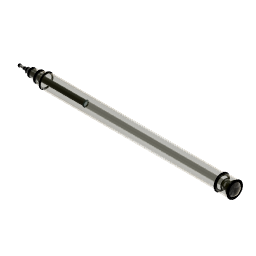
Pen_Model (Autodesk Fusion 360 design; units mm, degrees)
Autodesk Fusion 360 part; units mm, degrees
sketch "Sketch1" plane through (0, 0, 0) normal (0, 1, 0) x (1, 0, 0)
  line L0 (-51.000001, 0) -> (8, 0)
  line L1 (-50.999999, -0.45) -> (-51.000001, -0.5)
  line L2 (-51.000001, -0.5) -> (-48.500001, -0.5)
  line L3 (-48.500001, -0.5) -> (-47.077309, -0.848455)
  line L4 (-47.077309, -0.848455) -> (-47.077309, -0.95)
  line L5 (-41.000001, -1.35) -> (-41.000001, -1.175)
  arc A0 (-51.349999, 0) -> (-50.999999, -0.45) centre (-50.867104, 0.014474) ccw
  line L6 (-51.349999, 0) -> (-51.000001, 0)
  line L7 (-41.000001, -1.35) -> (-44.999999, -1.35)
  line L8 (-44.999999, -1.35) -> (-44.999999, -1.7)
  line L9 (-47.077309, -0.95) -> (-45.299999, -1.537888)
  line L10 (-45.299999, -1.537888) -> (-45.299999, -1.7)
  line L11 (-44.999999, -1.7) -> (-45.299999, -1.7)
  line L12 (-41.000001, -1.175) -> (19, -1.175)
  line L13 (19, -1.175) -> (19, 0)
  line L14 (19, 0) -> (8, 0)
  line L15 (-41.000001, -1.175) -> (-41.000001, 0)
  line L16 (-28.417661, -1.175) -> (-28.417661, 0)
  constraint horizontal L0
  constraint perpendicular L0 L1
  constraint perpendicular L1 L2
  constraint perpendicular L2 L4
  constraint parallel L0 L6
  constraint perpendicular L10 L11
  constraint perpendicular L12 L13
  constraint perpendicular L0 L15
revolve "Revolve1" add sketch "Sketch1" angle 360 about axis through (-51.000001, 0, 0) along (1, 0, 0) makes body 1
move_face "OffsetFaces1" offset -39 1 faces at (19, 0.344804, 0.639991) on bodies 1
sketch "Sketch2" plane through (-20, 0, 0) normal (1, 0, 0) x (0, 1, 0)
  circle A0 centre (0, 0) radius 1.175
sketch "Sketch3" plane through (-20, 0, 0) normal (1, 0, 0) x (0, 1, 0)
  circle A0 centre (0, 0) radius 1.173456
  circle A1 centre (0, 0) radius 1.111334
  constraint coincident A0.centre A1.centre
extrude "Extrude1" add sketch "Sketch3" along normal blind 69 bodies 1
fillet "Fillet1" radius 0.495 1 edges at (-51.000001, -0.180808, -0.466164) on bodies 1
sketch "Sketch4" plane through (0, 0, 0) normal (0, 1, 0) x (1, 0, 0)
  line L0 (-44.999999, -1.35) -> (-44.999999, -1.8)
  line L1 (-44.999999, -1.8) -> (-42.726678, -2.455447)
  line L2 (-42.726678, -2.455447) -> (-42.399999, -2.455447)
  line L3 (-42.399999, -2.455447) -> (-40.838311, -2.905716)
  line L4 (-40.838311, -2.905716) -> (43.000001, -2.905716)
  line L5 (43.000001, -2.905716) -> (43.000001, -3.5)
  line L6 (43.000001, -3.5) -> (49.000001, -3.5)
  line L7 (49.000001, -3.5) -> (49.000001, -1)
  line L8 (49.425851, -1) -> (49.425851, -3.5)
  line L9 (49.425851, -3.5) -> (49.000001, -3.5)
  line L10 (45.000001, 0) -> (45.000001, -2)
  line L11 (45.000001, -2) -> (48.000001, -2)
  line L12 (48.000001, -2) -> (48.000001, -2.6)
  line L13 (48.000001, -2.6) -> (49.000001, -2.6)
  line L14 (49.425851, 0) -> (49.425851, -1)
  arc A0 (49.425851, -2.989421) -> (50.690361, 0.022081) centre (46.648918, -0.052175) ccw
  line L15 (49, -1.173456) -> (49, 1.173456)
  line L16 (-20, 1.173456) -> (-20, -1.173456)
  line L17 (45.000001, 0) -> (45.000001, -2)
  line L18 (49.000001, 0) -> (50.690706, 0)
  line L19 (49.000001, 0) -> (49.000001, -2.6)
  line L20 (49.000001, 0) -> (45.000001, 0)
  constraint vertical L0
  constraint horizontal L2
  constraint parallel L1 L3
  constraint parallel L2 L4
  constraint perpendicular L4 L5
  constraint perpendicular L5 L6
  constraint perpendicular L6 L7
  constraint perpendicular L6 L8
  constraint perpendicular L7 L9
  constraint perpendicular L10 L11
  constraint perpendicular L11 L12
  constraint perpendicular L7 L13
  constraint perpendicular L13 L19
  constraint perpendicular L10 L20
revolve "Revolve2" add sketch "Sketch4" angle 360 about axis through (49.000001, 0, 0) along (1, 0, 0) separate body makes body 2
sketch "Sketch5" plane through (0, 0, 0) normal (0, 1, 0) x (1, 0, 0)
  line L0 (-20, 1.175) -> (-20, -1.175)
  line L1 (-41.000001, 1.175) -> (-41.000001, -1.175)
  line L2 (-41.000001, 1.35) -> (-41.000001, -1.35)
  line L3 (-44.999999, 1.35) -> (-44.999999, -1.35)
  line L4 (49, -1.173456) -> (49, 1.173456)
  line L5 (-20, 1.173456) -> (-20, -1.173456)
  line L6 (49.425851, 2.989421) -> (49.425851, -2.989421)
  line L7 (49.000001, 3.5) -> (49.000001, -3.5)
  line L8 (49.425851, 3.5) -> (49.425851, -3.5)
  line L9 (49.425851, 3.5) -> (49.425851, -3.5)
  line L10 (49.000001, 3.5) -> (49.000001, -3.5)
  line L11 (49.000001, 2.6) -> (49.000001, -2.6)
  line L12 (48.000001, 2.6) -> (48.000001, -2.6)
  line L13 (48.000001, 2) -> (48.000001, -2)
  line L14 (45.000001, 2) -> (45.000001, -2)
  line L15 (-44.999999, 1.7) -> (-44.999999, -1.7)
  line L16 (-45.299999, 1.7) -> (-45.299999, -1.7)
  line L17 (-44.999999, -1.7) -> (-44.999999, -1.73)
  line L18 (-44.999999, -1.73) -> (-41.853822, -2.38915)
  line L19 (-41.500001, -2.38915) -> (-39.838784, -2.811318)
  line L20 (49.000001, -3.5) -> (43.360207, -3.5)
  line L21 (43.360207, -3.5) -> (43.360207, -3.146671)
  line L22 (43.360207, -3.146671) -> (-38.519177, -3.146671)
  line L23 (-39.838784, -2.811318) -> (-38.519177, -3.146671)
  arc A0 (-41.853822, -2.38915) -> (-41.500001, -2.38915) centre (-41.676911, -2.258185) ccw
  arc A1 (-41.422098, -2.082604) -> (-41.676911, -2.126964) centre (-41.500001, -2.38915) ccw
  line L24 (-41.422098, -2.082604) -> (-39.760881, -2.504772)
  line L25 (-39.760881, -2.504772) -> (-38.479616, -2.830381)
  line L26 (43.676497, -2.830381) -> (-38.479616, -2.830381)
  line L27 (43.676497, -3.18371) -> (43.676497, -2.830381)
  line L28 (49.000001, -3.18371) -> (43.676497, -3.18371)
  line L29 (-41.676911, -2.126964) -> (-44.999999, -1.448771)
  dimension "d8" = -0.31629
  constraint parallel L15 L17
  constraint perpendicular L10 L20
  constraint perpendicular L20 L21
  constraint perpendicular L10 L22
  constraint parallel L19 L23
revolve "Revolve3" add sketch "Sketch5" angle 360 about axis through (-20, 0, 0) along (-1, 0, 0) bodies 1 2
